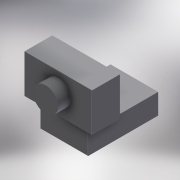
# Autodesk Inventor part: DK2 Camera
Saved by Autodesk Inventor 2017 (Build 210142000, 142)
## iProperties
Created: 2016-08-30
Part Number: DK2 Camera
Material: Generic
Document SubType Name: Modeling
Designer: Ali
Density: 1 g/cm^3
Appearance: Default
Author: Ali
Autodesk Inventor part; units mm, degrees
ref_plane "YZ Plane" through (0, 0, 0) normal (1, 0, 0) x (0, 1, 0)
ref_plane "XZ Plane" through (0, 0, 0) normal (0, 1, 0) x (-1, 0, 0)
ref_plane "XY Plane" through (0, 0, 0) normal (0, 0, 1) x (1, 0, 0)
sketch "Sketch1" plane through (0, 0, 0) normal (0, 0, 1) x (1, 0, 0)
  circle A0 centre (0, 17) radius 3.1 projected
  line L0 (19.75, -8) -> (-19.75, -8) projected
  line L1 (19.75, 33) -> (19.75, -8) projected
  line L2 (-19.75, 33) -> (19.75, 33) projected
  line L3 (-19.75, -8) -> (-19.75, 33) projected
  line L4 (-19.75, -8) -> (19.75, -8)
  line L5 (19.75, -8) -> (19.75, -17)
  line L6 (19.75, -17) -> (-19.75, -17)
  line L7 (-19.75, -17) -> (-19.75, -8)
  line L8 (-19.75, 33) -> (19.75, 33)
  line L9 (19.75, 33) -> (19.75, 41)
  line L10 (19.75, 41) -> (-19.75, 41)
  line L11 (-19.75, 41) -> (-19.75, 33)
  line L12 (-19.75, -10) -> (19.75, -10) projected
  point P0 (0, 0)
  dimension "d0" = 7
  dimension "d1" = 8
  constraints: 16 end point, 4 parallel, 2 horizontal, 2 perpendicular, 2 point on line
  measures "d0" distance between parallel lines of L6 L12
  measures "d1" distance between parallel lines of L10 L2
extrude "Extrusion1" add sketch "Sketch1" along normal blind 17 contours A0 | L5 L12 L7 L0 | L0 L3 L2 L1 | L2 L11 L10 L9 | L5 L6 L7 L12
sketch "Sketch2" plane through (0, 0, 17) normal (0, 0, 1) x (1, 0, 0)
  line L0 (-19.75, -17) -> (19.75, -17) projected
  line L1 (-15, -17) -> (15, -17)
  line L2 (15, -17) -> (15, -12)
  line L3 (15, -12) -> (-15, -12)
  line L4 (-15, -12) -> (-15, -17)
  line L5 (0, 0) -> (0, 11.2749)
  point P0 (0, -12)
  dimension "d4" = 30
  dimension "d5" = 5
  constraints: 10 end point, 2 parallel, 2 point on line, 1 horizontal, 1 midpoint, 1 perpendicular, 1 vertical
  measures "d4" distance of L2.end L3.end
  measures "d5" distance of L3.end L1.start
extrude "Extrusion2" add sketch "Sketch2" along normal blind 4.7
sketch "Sketch3" plane through (0, 0, 21.7) normal (0, 0, 1) x (1, 0, 0)
  line L0 (-15, -17) -> (15, -17) projected
  line L1 (15, -17) -> (15, -12) projected
  line L2 (15, -12) -> (-15, -12) projected
  line L3 (-15, -12) -> (-15, -17) projected
  line L4 (-28, -22) -> (28, -22)
  line L5 (28, -22) -> (28, 1)
  line L6 (28, 1) -> (-28, 1)
  line L7 (-28, 1) -> (-28, -22)
  line L8 (0, 0) -> (0, 8.1393)
  point P0 (0, 1)
  dimension "d8" = 56
  dimension "d9" = 23
  dimension "d10" = 5
  constraints: 10 end point, 2 parallel, 1 horizontal, 1 midpoint, 1 perpendicular, 1 point on line, 1 vertical
  measures "d8" distance of L4.start L4.end
  measures "d9" distance of L6.end L4.start
  measures "d10" distance between parallel lines of L0 L4
extrude "Extrusion3" add sketch "Sketch3" along normal blind 32 contours L3 L2 L1 L0 | L7 L6 L5 L4
sketch "Sketch4" plane through (-28, -22, 21.7) normal (0, -1, 0) x (1, 0, 0)
  circle A0 centre (28, 16.697) radius 10.25
  point P0 (28, -21.7)
  dimension "d13" = 20.5
  constraints: 1 centre point
  measures "d13" diameter of A0
extrude "Extrusion4" add sketch "Sketch4" along normal blind 10.5
fillet "Fillet1" radius 3 12 edges at (-28, -10.5, 53.7) (28, -10.5, 53.7) (28, -10.5, 21.7) (-28, -10.5, 21.7) (-28, -22, 37.7) (0, -22, 21.7) (0, -22, 53.7) (28, -22, 37.7) (28, 1, 37.7) (-28, 1, 37.7) (0, 1, 53.7) (0, 1, 21.7)
sketch "Sketch5" plane through (0, -32.5, 38.397) normal (0, -1, 0) x (1, 0, 0)
  circle A0 centre (0, 0) radius 10.25 projected
  circle A1 centre (0, 0) radius 7.1424
  point P0 (0, -38.397)
  constraints: 1 centre point
extrude "Extrusion5" cut sketch "Sketch5" against normal blind 1 contours A1
fillet "Fillet2" radius 1 2 edges at (15, -14.5, 17) (-15, -14.5, 17)
fillet "Fillet3" radius 4 2 edges at (0, 41, 0) (0, 41, 17)
body "Solid1"
